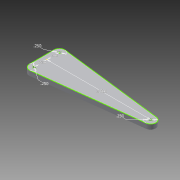
# Autodesk Inventor part: servo horn
Saved by Autodesk Inventor 2013 (Build 170138000, 138)
## iProperties
Created: 2013-09-17
Part Number: servo horn
Material: Aluminum 6061
Document SubType Name: Sheet Metal
Designer: Ian
Density: 2.71 g/cm^3
Sheet Metal Rule: Default
Mass: 7.96785 g
Surface Area: 24.6869 cm^2
Volume: 2.94017 cm^3
Author: Ian
Autodesk Inventor part; units mm, degrees
ref_plane "YZ Plane" through (0, 0, 0) normal (1, 0, 0) x (0, 1, 0)
ref_plane "XZ Plane" through (0, 0, 0) normal (0, 1, 0) x (-1, 0, 0)
ref_plane "XY Plane" through (0, 0, 0) normal (0, 0, 1) x (1, 0, 0)
sketch "Sketch1" plane through (0, 0, 0) normal (0, 1, 0) x (-1, 0, 0)
  arc A0 (-64.1227, 3.1133) -> (-63.8783, -3.1524) centre (-63.5, 0) ccw
  arc A1 (3.175, 7.62) -> (-0.3788, 10.7723) centre (0, 7.62) ccw
  arc A2 (-0.3783, -10.7724) -> (3.175, -7.62) centre (0, -7.62) ccw
  line L0 (-64.1227, 3.1133) -> (-0.3788, 10.7723)
  line L1 (-0.3783, -10.7724) -> (-63.8783, -3.1524)
  line L2 (3.175, 7.62) -> (3.175, -7.62)
  point P0 (0, 0)
  dimension "d0" = 7.62
  dimension "d1" = 7.62
  dimension "d2" = 63.5
  dimension "d3" = 6.35
  dimension "d4" = 6.35
  dimension "d5" = 6.35
  constraints: 6 end point, 6 point on circle, 4 tangent, 3 centre point, 3 coincident
  measures "d0" distance of point (0, 0) point (0, 7.62)
  measures "d1" distance of point (0, 0) point (0, -7.62)
  measures "d2" distance of point (0, 0) point (-63.5, 0)
  measures "d3" diameter of A0
  measures "d4" diameter of A1
  measures "d5" diameter of A2
extrude "Plate1" add sketch "Sketch1" against normal blind 3.048
hole "Hole1" at (0, 0, -7.62) at (0, 0, 7.62) at (63.5, 0, 0) direction (0, -1, 0) diameter 1.4732 end through all
equation "\"d13\" = Thickness"
equation "\"BendRadius\" = Thickness"
equation "\"BendReliefWidth\" = Thickness"
equation "\"BendReliefDepth\" = 0.5 * Thickness"
equation "\"CornerReliefSize\" = 4 * Thickness"
equation "\"MinimumRemnant\" = 2 * Thickness"
equation "\"TransitionRadius\" = BendRadius"
equation "\"JacobiRadiusSize\" = BendRadius"
equation "\"GapSize\" = Thickness"
equation "\"d7\" = BendRadius"
equation "\"Thickness\" = 3.048"
body "Solid1"
